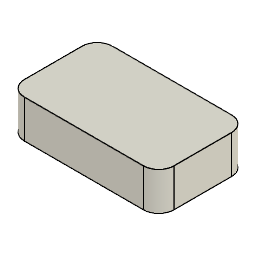
button cap v3 (Autodesk Fusion 360 design; units mm, degrees)
Autodesk Fusion 360 part; units mm, degrees
box "BoxPrimitive1" add length 11.5 width 19.5 height 4.97 placed x (0, 1, 0) y (-1, 0, 0) z (0, 0, 1) at (19.5059, 0, 0)
sketch "Sketch3" plane through (0, 0, 0) normal (0, 0, -1) x (1, 0, 0)
  line L0 (0.0059, -11.5) -> (19.5059, -11.5)
  line L1 (19.5059, -11.5) -> (19.5059, 0)
  line L2 (19.5059, 0) -> (0.0059, 0)
  line L3 (0.0059, 0) -> (0.0059, -11.5)
  line L4 (19.5059, -11.5) -> (0.0059, 0) construction
  line L5 (19.5059, 0) -> (0.0059, -11.5) construction
  line L6 (7.8559, -3.85) -> (11.6559, -3.85) construction
  line L7 (11.6559, -3.85) -> (11.6559, -7.65) construction
  line L8 (11.6559, -7.65) -> (7.8559, -7.65) construction
  line L9 (7.8559, -7.65) -> (7.8559, -3.85) construction
  line L10 (7.8559, -3.85) -> (11.6559, -7.65) construction
  line L11 (11.6559, -3.85) -> (7.8559, -7.65) construction
  circle A0 centre (9.7559, -5.75) radius 2.687
  point P0 (9.7559, -5.75)
  point P1 (9.7559, -5.75)
  dimension "d6" = 3.8
  constraint coincident L0.end L1.start
  constraint coincident L2.end L3.start
  constraint coincident L1.end L2.start
  constraint coincident L0.start L3.end
  constraint midpoint L5 P1
  constraint horizontal L6
  constraint perpendicular L6 L7
  constraint parallel L6 L8
  constraint parallel L7 L9
  constraint coincident L10 P1
  constraint coincident L11 P1
  constraint coincident P1 P0
  constraint equal L6 L9
  constraint coincident L6.start A0
  measures "d6" distance of L6.start L6.end
extrude "Extrude1" cut sketch "Sketch3" against normal blind 3 contours A0
fillet "Fillet1" radius 2 4 edges at (0.0059, 11.5, 2.485) (0.0059, 0, 2.485) (19.5059, 11.5, 2.485) (19.5059, 0, 2.485)
